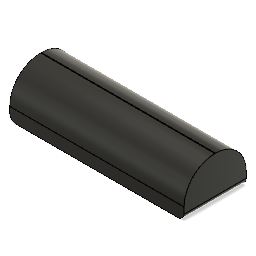
Suporte_Drible_Drt (Autodesk Fusion 360 archive; units mm, degrees)
design "Batente"
Autodesk Fusion 360 part; units mm, degrees
sketch "Esboço1" plane through (0, 0, 0) normal (0, 1, 0) x (1, 0, 0)
  line L0 (0, 0) -> (-56, 0)
  line L1 (-56, 0) -> (-56, -20)
  line L2 (-56, -20) -> (0, -20)
  line L3 (0, -20) -> (0, 0)
  dimension "d1" = 56
  dimension "d2" = 20
  constraint horizontal L0
  constraint vertical L1
  constraint horizontal L2
  constraint vertical L3
  constraint coincident L0.start L3.end
  measures "d1" distance of L0.start L0.end
  measures "d2" distance of L0.start L2.end
extrude "Extrusão1" add sketch "Esboço1" along normal blind 13.9
fillet "Arredondamento1" radius 9.9 2 edges at (-28, 13.9, 20) (-28, 13.9, 0)
fillet "Fillet2" radius 2 2 edges at (0, 0, 10) (-56, 0, 10)
